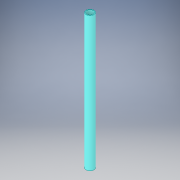
# Autodesk Inventor part: feet type 2 part 2 long
Saved by Autodesk Inventor 2018 (Build 220112000, 112)
## iProperties
Created: 2018-10-16
Part Number: feet type 2 part 2 long
Material: Fiber Glass
Document SubType Name: Modeling
Designer: freyja
Density: 1 g/cm^3
Appearance: Generic
Mass: 3.62685 g
Surface Area: 88.3217 cm^2
Volume: 3.62685 cm^3
Author: freyja
Autodesk Inventor part; units mm, degrees
ref_plane "YZ Plane" through (0, 0, 0) normal (1, 0, 0) x (0, 1, 0)
ref_plane "XZ Plane" through (0, 0, 0) normal (0, 1, 0) x (-1, 0, 0)
ref_plane "XY Plane" through (0, 0, 0) normal (0, 0, 1) x (1, 0, 0)
sketch "Sketch1" plane through (0, 0, 0) normal (0, 1, 0) x (-1, 0, 0)
  circle A0 centre (0, 0) radius 4.7625
  circle A1 centre (0, 0) radius 3.937
  dimension "d0" = 9.525
  dimension "d1" = 7.874
  constraints: 2 centre point, 2 coincident
  measures "d0" diameter of A0
  measures "d1" diameter of A1
extrude "Extrusion1" add sketch "Sketch1" along normal blind 160.7566
body "Solid1"
